Autodesk Inventor part; units mm, degrees
(part 2 of 2)
ref_plane "Work Plane8" through (-43.2823, 9.5041, -29.35) normal (0, 0, -1) x (-0.3802684, 0.9248762, 0)
ref_plane "Work Plane9" through (-49.9646, -8.4408, -26.85) normal (0, 0, 1) x (0.9248762, 0.3802684, 0)
extrude "Extrusion8" add sketch "Sketch4" against normal up to surface (7.65 mm away) contours L17 A121 L3 A120 | A120 L3 L18 L12 L17 | L17 L3 A121
ref_plane "Work Plane5" through (-23.1368, 52.6716, -30.5) normal (0, 0, 1) x (0.9993908, 0.0348995, 0)
extrude "Extrusion9" cut sketch "Sketch4" along normal blind 15.5 and the other way blind 4 contours L10 A120 L2 | A120 L10 L9 L11 L2
ref_plane "Work Plane1" through (-5, 81.9, -49.5) normal (0, 0, -1) x (0, 1, 0)
ref_plane "Work Plane2" through (-13.7357, 64.9938, -40) normal (-0.0348995, 0.9993908, 0) x (-0.9993908, -0.0348995, 0)
ref_plane "Work Plane3" through (-23.8, 0, -27.5) normal (0, 0, -1) x (0, 1, 0)
sketch "Sketch5" plane through (-13.7357, 64.9938, -40) normal (-0.0348995, 0.9993908, 0) x (-0.9993908, -0.0348995, 0)
  arc A0 (0, -0.2709) -> (0, -0.7291) centre (-5.245, -0.5) ccw projected
  arc A1 (0, -0.7291) -> (0, -0.2709) centre (5.245, -0.5) ccw projected
  circle A2 centre (-5.245, -0.5) radius 4.5 projected
  circle A3 centre (5.245, -0.5) radius 4.5 projected
  line L0 (0.5, 1.7467) -> (-0.5, 1.7467)
  line L1 (0.5, -2.7467) -> (-0.5, -2.7467)
  line L2 (0.5, 1.7467) -> (1.346, 1.7467)
  line L3 (-0.5, 1.7467) -> (-1.346, 1.7467)
  line L4 (-0.5, -2.7467) -> (-1.346, -2.7467)
  line L5 (0.5, -2.7467) -> (1.346, -2.7467)
  point P0 (-11.4591, 40)
  dimension "d30" = 1
  dimension "d31" = 1
  constraints: 12 end point, 8 point on circle, 3 point on line, 2 parallel, 1 horizontal
  measures "d30" distance of L0.start L0.end
  measures "d31" distance of L1.start L1.end
extrude "Extrusion14" cut sketch "Sketch5" along normal blind 2.5
extrude "Extrusion15" cut sketch "Sketch5" along normal through all contours A1 L2 A3 L5 A0 L4 A2 L3 | A0 L0 A1 | A0 A1 L1 | A2 | A3
sketch "Sketch8" plane through (-3, 81.4, 34.5) normal (0, 1, 0) x (1, 0, 0)
  line L0 (1.37, 83.5) -> (1.37, 67.5) projected
  line L1 (0.37, 83.5) -> (1.37, 83.5) projected
  line L2 (0.37, 67.5) -> (0.37, 83.5) projected
  line L3 (0.37, 67.5) -> (1.37, 67.5) projected
  line L4 (1.37, 83.5) -> (1.87, 83.5)
  line L5 (1.87, 83.5) -> (1.87, 67)
  line L6 (1.87, 67) -> (0.37, 67)
  line L7 (0.37, 67) -> (0.37, 67.5)
  point P0 (3, 34.5)
  dimension "d54" = 0.5
  dimension "d55" = 0.5
  constraints: 8 end point, 2 perpendicular, 1 horizontal, 1 parallel
  measures "d54" distance between parallel lines of L6 L3
  measures "d55" distance between parallel lines of L5 L0
extrude "Extrusion11" cut sketch "Sketch8" against normal through all
sketch "Sketch9" plane through (-27, 69.2958, -34.5) normal (-1, 0, 0) x (0, 0, 1)
  line L0 (-14.5, -3.7958) -> (1.5, -3.7958) projected
  line L1 (1.5, -3.7958) -> (1.5, 12.2042) projected
  line L2 (1.5, 12.2042) -> (-14.5, 12.2042) projected
  line L3 (-14.5, 12.2042) -> (-14.5, -3.7958) projected
  circle A0 centre (-12.475, 0.3442) radius 0.45 projected
  circle A1 centre (-4, 2.7042) radius 1.25 projected
  circle A2 centre (-12.475, 7.9642) radius 0.45 projected
  circle A3 centre (-12.475, 2.9642) radius 0.45 projected
  circle A4 centre (-12.475, 5.4242) radius 0.45 projected
  line L4 (-11.25, -2.986) -> (-11.25, 17.8025) construction
  line L5 (-14.5, 8.4142) -> (-12.025, 8.4142)
  line L6 (-12.025, 8.4142) -> (-12.025, -0.1058)
  line L7 (-12.025, -0.1058) -> (-14.5, -0.1058)
  line L8 (-14.5, -0.1058) -> (-14.5, 8.4142)
  ellipse E0 centre (-6, -2.6199) end of major axis (-0.75, -2.6199) minor radius 0.1832 (-5.7709, -2.803) -> (-6.2291, -2.803) ccw projected
  ellipse E1 centre (-6, -2.986) end of major axis (-0.75, -2.986) minor radius 0.1832 (-6.2291, -2.803) -> (-5.7709, -2.803) ccw projected
  ellipse E2 centre (-6, -2.6199) end of major axis (-1.5, -2.6199) minor radius 0.157 projected
  ellipse E3 centre (-6, -2.986) end of major axis (-1.5, -2.986) minor radius 0.157 projected
  point P0 (34.5, -69.2958)
  point P1 (-13.5, 8.4142)
  point P2 (-13.5, -3.9142)
  dimension "d58" = 0
  dimension "d59" = 0.775
  dimension "d60" = 0
  dimension "d61" = 0
  constraints: 10 end point, 2 parallel, 2 vertical, 1 horizontal, 1 perpendicular, 1 point on line, 3 other
  measures "d58" distance edge to line of A2 L6
  measures "d59" distance between parallel lines of L4 L6
  measures "d60" distance edge to line of A2 L5
  measures "d61" distance edge to line of A0 L7
extrude "Extrusion12" cut sketch "Sketch9" against normal up to surface (25.87 mm away) contours A3 | A4 | L3 L5 A2 L6 A0 L7 | A0 | A0 L6 L7 | L5 L6 A2 | A2
fillet "Fillet1" radius 2 3 edges at (-2.63, 73.45, -46.525) (-2.63, 77.71, -47.7625) (-2.63, 69.19, -47.7625)
sketch "Sketch10" plane through (0, 65.2958, 34.5) normal (1, 0, 0) x (0, 0, -1)
  line L0 (75.9, 14.1042) -> (80.4, 14.1042)
  line L1 (80.4, 14.1042) -> (80.4, 2.8042)
  line L2 (80.4, 2.8042) -> (75.9, 2.8042)
  line L3 (75.9, 2.8042) -> (75.9, 14.1042)
  line L4 (75.9, 14.1042) -> (75.9, 16.2042)
  line L5 (80.4, 16.2042) -> (80.4, 14.1042)
  line L6 (67.5, 16.2042) -> (67.5, 0.2042) projected
  line L7 (67.5, 0.2042) -> (83.5, 0.2042) projected
  line L8 (83.5, 0.2042) -> (83.5, 16.2042) projected
  line L9 (83.5, 16.2042) -> (67.5, 16.2042) projected
  line L10 (79.9, 13.1042) -> (79.9, 9.6042) projected
  line L11 (79.9, 9.6042) -> (76.4, 9.6042) projected
  line L12 (76.4, 9.6042) -> (76.4, 13.1042) projected
  line L13 (76.4, 13.1042) -> (79.9, 13.1042) projected
  line L14 (76.4, 6.8042) -> (79.9, 6.8042) projected
  line L15 (79.9, 6.8042) -> (79.9, 3.3042) projected
  line L16 (79.9, 3.3042) -> (76.4, 3.3042) projected
  line L17 (76.4, 3.3042) -> (76.4, 6.8042) projected
  circle A0 centre (81.475, 4.3442) radius 0.45 projected
  circle A1 centre (73, 6.7042) radius 1.25 projected
  circle A2 centre (81.475, 11.9642) radius 0.45 projected
  circle A3 centre (81.475, 6.9642) radius 0.45 projected
  circle A4 centre (81.475, 9.4242) radius 0.45 projected
  point P0 (34.5, -65.2958)
  dimension "d151" = 0.5
  dimension "d152" = 0.5
  dimension "d153" = 0.5
  constraints: 12 end point, 2 parallel, 2 perpendicular, 1 collinear, 1 horizontal
  measures "d151" distance between parallel lines of L10 L1
  measures "d152" distance between parallel lines of L3 L12
  measures "d153" distance between parallel lines of L2 L16
extrude "Extrusion13" cut sketch "Sketch10" against normal up to surface (1.13 mm away) contours L4 L9 L5 L0 | L0 L1 L2 L3 | L10 L11 L12 L13 | L14 L15 L16 L17
ref_plane "Work Plane6" through (-13.7357, 64.9938, -40) normal (-0.0348995, 0.9993908, 0) x (-0.9993908, -0.0348995, 0)
sketch "Sketch12" plane through (-13.7357, 64.9938, -40) normal (-0.0348995, 0.9993908, 0) x (-0.9993908, -0.0348995, 0)
  circle A0 centre (9.6, 6.0491) radius 0.75 projected
  circle A1 centre (0, -6.5) radius 0.75 projected
  circle A2 centre (-9.6, 6.0491) radius 0.75 projected
  point P0 (-11.4591, 40)
hole "Hole2" at (-23.3298, 64.6588, -33.9509) at (-13.7357, 64.9938, -46.5) at (-4.1415, 65.3288, -33.9509) direction (-0.0348995, 0.9993908, 0) diameter 2.5 depth 5 counterbore diameter 3 counterbore depth 1
sketch "Sketch16" plane through (-27, 69.2958, -34.5) normal (-1, 0, 0) x (0, 0, 1)
  line L0 (-12.025, 8.4142) -> (-12.025, -0.1058) projected
  line L1 (-14.5, -0.1058) -> (-14.5, 8.4142) projected
  line L2 (0, 0) -> (0, 17) projected
  line L3 (-15.5, -4) -> (-15.5, 17) projected
  line L4 (7.65, -4) -> (7.65, 0) projected
  line L5 (0, 0) -> (7.65, 0) projected
  line L6 (-12.025, 8.4142) -> (0, 8.5)
  line L7 (-13.25, -0.1058) -> (-12.025, -0.1058) projected
  line L8 (-1.5, -1.6205) -> (-1.5, 20.3536) projected
  line L9 (-15.5, -4) -> (7.65, -4) projected
  line L10 (0, 17) -> (-15.5, 17) projected
  line L11 (-12.025, -0.1058) -> (-14.5, -0.1058) projected
  line L12 (-14.5, 8.4142) -> (-12.025, 8.4142) projected
  line L13 (-12.025, 8.4142) -> (-12.025, -0.1058) projected
  line L14 (-12.025, -0.1058) -> (-10.025, -2.1058) projected
  line L15 (0, 0) -> (-12.025, -0.1058)
  point P0 (34.5, -69.2958)
  point P1 (-11.025, -0.1058)
  point P2 (-1.5, 8.4893)
  point P3 (-12.025, 8.4142)
  point P4 (-13.25, -0.1058)
  constraints: 4 end point, 1 midpoint
extrude "Extrusion16" cut sketch "Sketch16" against normal blind 2 contours L6 L8 L15 L0 | L6 L2 L15 L8
sketch "Sketch15" plane through (-26.7898, 86.3358, -34.5) normal (-0.18665, 0.9824265, 0) x (0.9824265, 0.18665, 0)
  circle A0 centre (12.4464, 12.1288) radius 3
  circle A1 centre (2.786, 12.1288) radius 3
  line L0 (-0.214, 0) -> (-0.214, 15.5) projected
  ellipse E0 centre (7.1395, 6) end of major axis (2.5865, 6) minor radius 4.5 (11.0846, 8.2467) -> (11.0846, 3.7533) ccw projected
  ellipse E1 centre (17.7533, 6) end of major axis (13.2002, 6) minor radius 4.5 (13.8082, 3.7533) -> (13.8082, 8.2467) ccw projected
  point P0 (10.2044, -34.5)
  dimension "d94" = 6
  dimension "d95" = 6
  dimension "d159" = 5.3069
  dimension "d160" = 5.3069
  dimension "d162" = 0
  constraints: 2 centre point, 1 tangent, 3 other
  measures "d94" diameter of A0
  measures "d95" diameter of A1
  measures "d159" horizontal distance of A0.centre point (17.753, 6)
  measures "d160" horizontal distance of A0.centre point (7.14, 6)
  measures "d162" vertical distance of A1.centre A0.centre
hole "Hole3" at (-24.0527, 86.8558, -46.6288) at (-14.5621, 88.6589, -46.6288) direction (0.18665, -0.9824265, 0) diameter 4 depth 4 counterbore diameter 4.5 counterbore depth 0.5
sketch "Sketch17" plane through (-27, 65.2958, -50) normal (-1, 0, 0) x (0, 0, 1)
  line L0 (0, 12.4465) -> (8, 12.4465)
  line L1 (8, 12.4465) -> (8, 17.4465)
  line L2 (8, 17.4465) -> (0, 17.4465)
  line L3 (0, 17.4465) -> (0, 12.4465)
  line L4 (15.5, 12.5) -> (15.5, 12.5) projected
  line L5 (8, 17.4465) -> (0, 12.4465)
  line L6 (0, 17.4465) -> (8, 12.4465)
  point P0 (50, -65.2958)
  point P1 (3.475, 12.4142)
  point P2 (4, 14.9465)
  point P3 (3.475, 12.4142)
  dimension "d107" = 8
  dimension "d108" = 5
  constraints: 12 end point, 2 parallel, 1 horizontal, 1 midpoint, 1 perpendicular, 2 other
  measures "d107" distance of L1.end L2.end
  measures "d108" distance of L0.end L1.end
hole "Hole4" at (-27, 80.2423, -46) direction (1, 0, 0) diameter 4 depth 4.5 counterbore diameter 4.5 counterbore depth 0.5
ref_plane "Work Plane7" through (-13.7357, 64.9938, -40) normal (-0.0348995, 0.9993908, 0) x (-0.9993908, -0.0348995, 0)
sketch "Sketch18" plane through (-13.7357, 64.9938, -40) normal (-0.0348995, 0.9993908, 0) x (-0.9993908, -0.0348995, 0)
  circle A0 centre (0, -6.5) radius 0.75 projected
  circle A1 centre (9.6, 6.0491) radius 0.75 projected
  circle A2 centre (-9.6, 6.0491) radius 0.75 projected
  line L0 (-12.325, 5.5) -> (-12.325, -4.5) projected
  arc A3 (-12.325, -4.5) -> (-8.325, -8.5) centre (-8.325, -4.5) ccw projected
  line L1 (-8.325, -8.5) -> (8.325, -8.5) projected
  arc A4 (8.325, -8.5) -> (12.325, -4.5) centre (8.325, -4.5) ccw projected
  line L2 (12.325, -4.5) -> (12.325, 5.5) projected
  arc A5 (12.325, 5.5) -> (9.325, 8.5) centre (9.325, 5.5) ccw projected
  line L3 (9.325, 8.5) -> (-9.325, 8.5) projected
  arc A6 (-9.325, 8.5) -> (-12.325, 5.5) centre (-9.325, 5.5) ccw projected
  arc A7 (0, -0.2709) -> (0, -0.7291) centre (-5.245, -0.5) ccw projected
  arc A8 (0, -0.7291) -> (0, -0.2709) centre (5.245, -0.5) ccw projected
  line L4 (3, 8.5) -> (-3, 8.5)
  line L5 (-3, 8.5) -> (-3, 7.5)
  line L6 (-3, 7.5) -> (3, 7.5)
  line L7 (3, 7.5) -> (3, 8.5)
  line L8 (-13.7379, 10.65) -> (-10.24, 10.65) projected
  line L9 (3, 8.5) -> (3, 10.65)
  line L10 (-3, 8.5) -> (-3, 10.65)
  line L11 (-3, 10.65) -> (3, 10.65)
  point P0 (-11.4591, 40)
  dimension "d116" = 9.325
  dimension "d117" = 9.325
  dimension "d118" = 1
  dimension "d173" = 2.15
  dimension "d174" = 6
  constraints: 14 end point, 3 perpendicular, 3 point on line, 2 parallel, 1 horizontal, 1 vertical
  measures "d116" distance between parallel lines of L7 L2
  measures "d117" distance between parallel lines of L5 L0
  measures "d118" distance between parallel lines of L4 L6
  measures "d173" distance between parallel lines of L11 L4
  measures "d174" distance of L5.end L6.end
extrude "Extrusion17" cut sketch "Sketch18" along normal blind 10 contours L10 L11 L9 L3 | L3 L7 L6 L5
sketch "Sketch19" plane through (-23.8, 69.2958, -17.65) normal (0, 1, 0) x (1, 0, 0)
  circle A0 centre (4, 4.55) radius 2.25 projected
  circle A1 centre (4, 4.55) radius 3.5
  ellipse E0 centre (0.3082, 16.3009) end of major axis (-0.9425, 16.3009) minor radius 1.25 (-0.8154, 16.85) -> (1.4319, 16.85) ccw projected
  line L0 (14.5915, -37.4) -> (0, -37.4) projected
  line L1 (0, -37.4) -> (0, -52.15) projected
  line L2 (17.8, -52.15) -> (0, -52.15) projected
  line L3 (17.8, 16.85) -> (17.8, -52.15) projected
  line L4 (-3.2, 9.2) -> (0, 9.2) projected
  line L5 (0, 0) -> (0, 9.2) projected
  line L6 (0, 0) -> (14.5915, 0) projected
  line L7 (6.9123, 11.7) -> (0, 5.2)
  line L8 (6.9123, 14.85) -> (0, 9.2)
  line L9 (6.0862, 11.7) -> (6.0862, 15.35)
  line L10 (12.9159, 14.85) -> (12.9159, 11.7) projected
  line L11 (12.9159, 11.7) -> (6.9123, 11.7) projected
  line L12 (6.9123, 11.7) -> (6.9123, 14.85) projected
  line L13 (6.9123, 14.85) -> (12.9159, 14.85) projected
  line L14 (1.4319, 16.85) -> (17.8, 16.85) projected
  line L15 (-1.2, 16.85) -> (-0.8154, 16.85) projected
  line L16 (-3.2, 16.85) -> (-1.2, 16.85) projected
  line L17 (-3.2, 16.85) -> (-3.2, 9.2) projected
  line L18 (14.5915, 0) -> (14.5915, -37.4) projected
  point P0 (23.8, -17.65)
  point P1 (5.0862, 12.5932)
  point P2 (6.0862, 15.35)
  dimension "d121" = 7
  dimension "d122" = 4
  constraints: 6 end point, 2 point on line, 1 centre point, 1 coincident, 1 vertical, 1 other
  measures "d121" diameter of A1
  measures "d122" distance of L4.end L7.end
extrude "Extrusion18" cut sketch "Sketch19" against normal blind 2 contours L7 A1 | A1 L7 L5 L8 L12 | L12 L13 L10 L11 picked at (1.5777, 6.7815)
mirror "Mirror2" about plane through (0, 0, 0) normal (0, 0, 1) of "Extrusion7", "Extrusion8", "Extrusion9", "Extrusion14", "Extrusion15", "Extrusion11", "Extrusion12", "Fillet1", "Extrusion13", "Hole2", "Extrusion16", "Hole3", "Hole4", "Extrusion17", "Extrusion18"
sketch "Sketch20" plane through (0, 81.4, -50) normal (1, 0, 0) x (0, 0, -1)
  line L0 (-100, 0.5) -> (-100, 15.6) projected
  line L1 (-100, 0.5) -> (-82.5, 0.5) projected
  circle A0 centre (-82.5, 4) radius 3.5 projected
  line L2 (-82.5, 0.5) -> (-66.25, 0.5) projected
  circle A1 centre (-66.25, 4) radius 3.5 projected
  line L3 (-66.25, 0.5) -> (-50, 0.5) projected
  circle A2 centre (-50, 4) radius 3.5 projected
  line L4 (-50, 0.5) -> (-33.75, 0.5) projected
  circle A3 centre (-33.75, 4) radius 3.5 projected
  line L5 (-33.75, 0.5) -> (-17.5, 0.5) projected
  circle A4 centre (-17.5, 4) radius 3.5 projected
  line L6 (-17.5, 0.5) -> (0, 0.5) projected
  line L7 (0, 15.6) -> (0, 0.5) projected
  line L8 (-100, 15.6) -> (0, 15.6) projected
  point P0 (-50, -81.4)
  constraints: 5 vertical alignment
hole "Hole5" at (0, 85.4, 32.5) at (0, 85.4, 16.25) at (0, 85.4, 0) at (0, 85.4, -16.25) at (0, 85.4, -32.5) direction (-1, 0, 0) diameter 2.459 depth 8.8 countersink diameter 3.5 countersink angle 90 thread size "M3x0.5" class "6H" standard "ISO Metric profile"
sketch "Sketch22" plane through (-23.8, 69.2958, -17.65) normal (0, 1, 0) x (1, 0, 0)
  circle A0 centre (14.3, -42.6439) radius 1.2295 projected
  circle A1 centre (3.7, 4.6) radius 2 projected
  circle A2 centre (7.1, -42.6439) radius 1.2295 projected
  circle A3 centre (11.3, 3.8) radius 2 projected
  circle A4 centre (11.3, 4.6) radius 2 projected
  circle A5 centre (14.3, -42.6439) radius 1.2295 projected
  point P0 (23.8, -17.65)
  point P1 (12.7, 4.55)
hole "Hole6" at (-16.7, 69.2958, 24.9939) at (-9.5, 69.2958, 24.9939) at (-20.1, 69.2958, -22.25) at (-12.5, 69.2958, -21.45) direction (0, -1, 0) diameter 3.4 depth 8.8 countersink diameter 7 countersink angle 90 clearance for "Countersunk Flat Head Screw ISO 2009/7046" size "M3" standard "ISO"
body "Solid2"
